Autodesk Fusion 360 part; units mm, degrees
(part 18 of 25)
  arc A5421 (73.9284, 22.9292) -> (73.8069, 23.2226) centre (73.8676, 23.0759) ccw
  line L1960 (79.2155, 20.3327) -> (79.2246, 20.3106)
  line L1961 (74.5699, 19.5453) -> (75.2188, 19.8141)
  arc A5422 (73.3311, 22.6949) -> (73.1066, 22.9194) centre (73.2189, 22.8072) ccw
  arc A5423 (73.8677, 23.2346) -> (73.8677, 22.9171) centre (73.8677, 23.0758) ccw
  arc A5424 (71.3073, 21.6383) -> (71.6007, 21.5168) centre (71.454, 21.5776) ccw
  arc A5425 (75.5687, 20.3714) -> (75.862, 20.2499) centre (75.7154, 20.3106) ccw
  line L1962 (71.628, 21.9976) -> (71.628, 24.4198)
  arc A5426 (81.0116, 19.692) -> (81.1331, 19.3986) centre (81.0724, 19.5453) ccw
  arc A5427 (72.6123, 21.6617) -> (72.2948, 21.6617) centre (72.4536, 21.6617) ccw
  arc A5428 (74.5699, 22.9171) -> (74.5699, 23.2346) centre (74.5699, 23.0758) ccw
  line L1963 (81.0723, 19.5453) -> (81.292, 19.6363)
  arc A5429 (73.1581, 18.4326) -> (73.2796, 18.1393) centre (73.2189, 18.2859) ccw
  arc A5430 (75.8712, 20.272) -> (75.5778, 20.3934) centre (75.7245, 20.3327) ccw
  arc A5431 (72.39, 25.2413) -> (72.39, 25.5588) centre (72.39, 25.4001) ccw
  arc A5432 (73.0125, 26.7442) -> (72.788, 26.5196) centre (72.9002, 26.6319) ccw
  arc A5433 (74.9617, 29.4567) -> (74.6442, 29.4567) centre (74.8029, 29.4567) ccw
  line L1964 (71.8797, 24.1681) -> (72.39, 24.1681)
  arc A5434 (71.7747, 21.9369) -> (71.4813, 22.0584) centre (71.628, 21.9977) ccw
  arc A5435 (72.2312, 24.1681) -> (72.5487, 24.1681) centre (72.3899, 24.1681) ccw
  arc A5436 (73.7806, 25.9103) -> (73.4631, 25.9103) centre (73.6218, 25.9103) ccw
  arc A5437 (73.9284, 18.408) -> (73.8069, 18.7014) centre (73.8676, 18.5547) ccw
  arc A5438 (79.2554, 18.0447) -> (79.4799, 17.8201) centre (79.3676, 17.9324) ccw
  arc A5439 (73.5177, 27.2925) -> (73.2002, 27.2925) centre (73.359, 27.2925) ccw
  arc A5440 (72.2312, 25.4) -> (72.5487, 25.4) centre (72.3899, 25.4) ccw
  arc A5441 (71.8797, 26.7906) -> (71.8797, 26.4731) centre (71.8797, 26.6319) ccw
  line L1965 (72.8653, 17.9324) -> (71.314, 17.9324)
  arc A5442 (74.6442, 28.9826) -> (74.9617, 28.9826) centre (74.8029, 28.9826) ccw
  arc A5443 (80.4308, 18.408) -> (80.3093, 18.7014) centre (80.3701, 18.5547) ccw
  arc A5444 (79.6605, 18.4326) -> (79.782, 18.1393) centre (79.7212, 18.2859) ccw
  line L1966 (72.39, 24.1681) -> (72.9003, 24.1681)
  arc A5445 (71.314, 18.0911) -> (71.314, 17.7736) centre (71.314, 17.9323) ccw
  arc A5446 (69.9162, 19.5548) -> (69.6917, 19.3303) centre (69.804, 19.4426) ccw
  line L1967 (74.803, 29.4567) -> (74.93, 29.5837)
  arc A5447 (72.5487, 26.6319) -> (72.2312, 26.6319) centre (72.3899, 26.6319) ccw
  arc A5448 (71.4692, 21.9976) -> (71.7867, 21.9976) centre (71.6279, 21.9976) ccw
  arc A5449 (75.0423, 29.4714) -> (74.8177, 29.6959) centre (74.93, 29.5837) ccw
  line L1968 (74.93, 29.5837) -> (75.2, 29.3137)
  arc A5450 (72.39, 24.3269) -> (72.39, 24.0094) centre (72.39, 24.1682) ccw
  arc A5451 (71.7867, 24.4198) -> (71.4692, 24.4198) centre (71.6279, 24.4198) ccw
  line L1969 (71.314, 17.9324) -> (69.8039, 19.4425)
  arc A5452 (74.5699, 18.3959) -> (74.5699, 18.7134) centre (74.5699, 18.5547) ccw
  arc A5453 (75.158, 18.1393) -> (75.2795, 18.4326) centre (75.2188, 18.2859) ccw
  arc A5454 (73.7342, 24.7775) -> (73.5096, 25.002) centre (73.6219, 24.8897) ccw
  arc A5455 (71.4692, 26.3802) -> (71.7867, 26.3802) centre (71.6279, 26.3802) ccw
  line L1970 (74.803, 28.9826) -> (74.803, 29.4567)
  line L1971 (71.628, 26.3802) -> (71.628, 26.797)
  line L1972 (71.454, 21.5775) -> (71.628, 21.9976)
  line L1973 (75.2188, 18.2859) -> (74.5699, 18.5547)
  line L1974 (72.9003, 26.6319) -> (72.39, 26.6319)
  arc A5456 (79.3677, 17.7736) -> (79.3677, 18.0911) centre (79.3677, 17.9323) ccw
  arc A5457 (72.9003, 24.0094) -> (72.9003, 24.3269) centre (72.9003, 24.1682) ccw
  arc A5458 (71.2018, 17.8201) -> (71.4263, 18.0447) centre (71.3141, 17.9324) ccw
  arc A5459 (69.6917, 19.5548) -> (69.9162, 19.3303) centre (69.804, 19.4426) ccw
  line L1975 (72.39, 24.1681) -> (72.39, 25.4)
  line L1976 (70.0659, 20.1895) -> (71.454, 21.5775)
  line L1977 (71.8797, 26.6319) -> (71.628, 26.3802)
  arc A5460 (74.9497, 28.9219) -> (74.6563, 29.0434) centre (74.803, 28.9827) ccw
  line L1978 (79.7212, 18.2859) -> (79.3677, 17.9324)
  line L1979 (72.39, 26.6319) -> (72.39, 25.4)
  arc A5461 (72.753, 18.0447) -> (72.9775, 17.8201) centre (72.8653, 17.9324) ccw
  arc A5462 (70.1781, 19.5923) -> (69.9536, 19.8168) centre (70.0658, 19.7046) ccw
  arc A5463 (69.9536, 20.3017) -> (70.1781, 20.0772) centre (70.0659, 20.1895) ccw
  arc A5464 (71.5662, 21.4653) -> (71.3417, 21.6898) centre (71.454, 21.5776) ccw
  arc A5465 (70.2246, 20.1895) -> (69.9071, 20.1895) centre (70.0658, 20.1895) ccw
  arc A5466 (72.2313, 25.4) -> (72.5488, 25.4) centre (72.3901, 25.4) ccw
  arc A5467 (79.8335, 18.1737) -> (79.609, 18.3982) centre (79.7212, 18.2859) ccw
  arc A5468 (74.4823, 28.6233) -> (74.7757, 28.5018) centre (74.629, 28.5626) ccw
  line L1980 (73.6219, 25.4) -> (72.39, 25.4)
  arc A5469 (72.9003, 26.4731) -> (72.9003, 26.7906) centre (72.9003, 26.6319) ccw
  arc A5470 (73.4712, 27.1803) -> (73.2467, 27.4048) centre (73.359, 27.2926) ccw
  arc A5471 (73.0982, 26.8243) -> (72.9767, 27.1177) centre (73.0375, 26.971) ccw
  arc A5472 (73.8677, 18.7134) -> (73.8677, 18.3959) centre (73.8677, 18.5547) ccw
  arc A5473 (75.4601, 17.8201) -> (75.6846, 18.0447) centre (75.5724, 17.9324) ccw
  arc A5474 (80.3701, 18.7134) -> (80.3701, 18.3959) centre (80.3701, 18.5547) ccw
  arc A5475 (75.5723, 18.0911) -> (75.5723, 17.7736) centre (75.5723, 17.9323) ccw
  line L1981 (72.39, 25.4) -> (73.6219, 25.4)
  line L1982 (75.5723, 17.9324) -> (75.2188, 18.2859)
  line L1983 (77.47, 29.5837) -> (77.74, 29.3137)
  line L1984 (77.74, 29.3137) -> (78.3889, 29.0449)
  line L1985 (80.2955, 29.6574) -> (80.4879, 29.5176)
  arc A5476 (80.1832, 29.5452) -> (80.4077, 29.7697) centre (80.2955, 29.6575) ccw
  arc A5477 (78.3281, 28.8982) -> (78.4496, 29.1916) centre (78.3889, 29.0449) ccw
  line L1986 (81.28, 29.2989) -> (81.28, 31.75)
  arc A5478 (72.39, 26.4731) -> (72.39, 26.7906) centre (72.39, 26.6319) ccw
  arc A5479 (73.4631, 24.8897) -> (73.7806, 24.8897) centre (73.6218, 24.8897) ccw
  line L1987 (75.8489, 29.0449) -> (76.5511, 29.0449)
  arc A5480 (72.39, 25.5588) -> (72.39, 25.2413) centre (72.39, 25.4001) ccw
  arc A5481 (73.4631, 25.4) -> (73.7806, 25.4) centre (73.6218, 25.4) ccw
  arc A5482 (72.39, 26.7906) -> (72.39, 26.4731) centre (72.39, 26.6319) ccw
  arc A5483 (73.6219, 25.2413) -> (73.6219, 25.5588) centre (73.6219, 25.4001) ccw
  arc A5484 (77.6278, 29.2014) -> (77.8523, 29.4259) centre (77.74, 29.3136) ccw
  arc A5485 (71.628, 26.9558) -> (71.628, 26.6382) centre (71.628, 26.797) ccw
  line L1988 (74.629, 28.5625) -> (74.803, 28.9826)
  line L1989 (76.5511, 29.0449) -> (77.2, 29.3137)
  arc A5486 (77.8008, 29.4603) -> (77.6793, 29.167) centre (77.74, 29.3137) ccw
  arc A5487 (79.0304, 29.1916) -> (79.1519, 28.8982) centre (79.0911, 29.0449) ccw
  arc A5488 (73.6219, 25.2412) -> (73.6219, 25.5587) centre (73.6219, 25.4) ccw
  arc A5489 (81.28, 31.9087) -> (81.28, 31.5912) centre (81.28, 31.75) ccw
  arc A5490 (81.1362, 29.1421) -> (81.1859, 29.4557) centre (81.1611, 29.2989) ccw
  arc A5491 (72.788, 24.2804) -> (73.0125, 24.0558) centre (72.9003, 24.1681) ccw
  arc A5492 (72.39, 25.5587) -> (72.39, 25.2412) centre (72.39, 25.4) ccw
  arc A5493 (72.39, 25.5588) -> (72.39, 25.2413) centre (72.39, 25.4001) ccw
  arc A5494 (71.7867, 26.797) -> (71.4692, 26.797) centre (71.6279, 26.797) ccw
  arc A5495 (73.2002, 27.2925) -> (73.5177, 27.2925) centre (73.359, 27.2925) ccw
  line L1990 (79.0911, 29.0449) -> (79.74, 29.3137)
  arc A5496 (78.3889, 29.2037) -> (78.3889, 28.8862) centre (78.3889, 29.045) ccw
  arc A5497 (81.1212, 29.2989) -> (81.4387, 29.2989) centre (81.2799, 29.2989) ccw
  arc A5498 (75.0423, 29.6959) -> (74.8177, 29.4714) centre (74.93, 29.5836) ccw
  line L1991 (81.28, 31.75) -> (81.28, 29.2989)
  arc A5499 (81.4388, 31.75) -> (81.1213, 31.75) centre (81.2801, 31.75) ccw
  arc A5500 (75.7881, 28.8982) -> (75.9096, 29.1916) centre (75.8488, 29.0449) ccw
  arc A5501 (74.7412, 28.4503) -> (74.5167, 28.6748) centre (74.629, 28.5626) ccw
  arc A5502 (74.6907, 29.5689) -> (74.9153, 29.3444) centre (74.803, 29.4566) ccw
  line L1992 (72.39, 25.4) -> (72.39, 26.6319)
  arc A5503 (81.1611, 29.4577) -> (81.1611, 29.1401) centre (81.1611, 29.2989) ccw
  arc A5504 (71.992, 26.5196) -> (71.7675, 26.7441) centre (71.8798, 26.6319) ccw
  arc A5505 (71.5157, 26.4924) -> (71.7403, 26.2679) centre (71.628, 26.3802) ccw
  arc A5506 (73.5096, 25.798) -> (73.7342, 26.0225) centre (73.6219, 25.9103) ccw
  line L1993 (72.9003, 24.1681) -> (73.6219, 24.8897)
  arc A5507 (72.5488, 26.6319) -> (72.2313, 26.6319) centre (72.3901, 26.6319) ccw
  arc A5508 (81.28, 31.5912) -> (81.28, 31.9087) centre (81.28, 31.75) ccw
  arc A5509 (73.2467, 27.4048) -> (73.4712, 27.1803) centre (73.359, 27.2926) ccw
  line L1994 (73.359, 27.2925) -> (74.629, 28.5625)
  arc A5510 (72.6174, 26.6382) -> (72.6174, 26.9558) centre (72.6174, 26.797) ccw
  line L1995 (73.6219, 25.4) -> (73.6219, 25.9103)
  arc A5511 (72.5566, 26.9437) -> (72.6781, 26.6503) centre (72.6174, 26.797) ccw
  arc A5512 (72.9252, 27.0833) -> (73.1497, 26.8588) centre (73.0375, 26.9711) ccw
  line L1996 (80.9261, 29.3361) -> (81.1611, 29.2989)
  line L1997 (73.0375, 26.971) -> (73.359, 27.2925)
  line L1998 (71.628, 26.797) -> (72.6174, 26.797)
  arc A5513 (73.7806, 25.4) -> (73.4631, 25.4) centre (73.6218, 25.4) ccw
  line L1999 (73.6219, 24.8897) -> (73.6219, 25.4)
  arc A5514 (72.5488, 25.4) -> (72.2313, 25.4) centre (72.3901, 25.4) ccw
  arc A5515 (72.2313, 25.4) -> (72.5488, 25.4) centre (72.3901, 25.4) ccw
  arc A5516 (80.3019, 29.8755) -> (80.0773, 29.651) centre (80.1896, 29.7633) ccw
  line L2000 (80.1896, 29.7633) -> (80.2955, 29.6574)
  arc A5517 (80.3888, 29.7859) -> (80.2021, 29.529) centre (80.2954, 29.6575) ccw
  line L2001 (73.6219, 25.9103) -> (72.9003, 26.6319)
  line L2002 (72.6174, 26.797) -> (73.0375, 26.971)
  line L2003 (72.39, 26.6319) -> (71.8797, 26.6319)
  arc A5518 (77.5823, 29.6959) -> (77.3577, 29.4714) centre (77.47, 29.5837) ccw
  arc A5519 (82.9051, 30.4072) -> (82.6031, 30.5054) centre (82.7541, 30.4563) ccw
  line L2004 (81.28, 29.2989) -> (81.3989, 29.2989)
  arc A5520 (81.1213, 29.2989) -> (81.4388, 29.2989) centre (81.2801, 29.2989) ccw
  arc A5521 (81.9092, 29.2586) -> (81.8111, 29.5606) centre (81.8602, 29.4096) ccw
  line L2005 (81.3989, 29.2989) -> (81.6339, 29.3361)
  arc A5522 (81.3989, 29.1401) -> (81.3989, 29.4577) centre (81.3989, 29.2989) ccw
  arc A5523 (79.6277, 29.4259) -> (79.8522, 29.2014) centre (79.74, 29.3137) ccw
  line L2006 (81.1611, 29.2989) -> (81.28, 29.2989)
  arc A5524 (80.6278, 29.2682) -> (80.7719, 29.5511) centre (80.6998, 29.4097) ccw
  arc A5525 (75.2608, 29.4603) -> (75.1393, 29.167) centre (75.2001, 29.3137) ccw
  arc A5526 (81.4388, 31.75) -> (81.1213, 31.75) centre (81.2801, 31.75) ccw
  arc A5527 (82.4441, 33.3886) -> (82.701, 33.5752) centre (82.5726, 33.4819) ccw
  arc A5528 (81.6091, 34.0071) -> (81.6587, 34.3207) centre (81.6339, 34.1639) ccw
  line L2007 (82.7541, 33.0437) -> (82.6806, 33.2699)
  arc A5529 (80.877, 29.1851) -> (80.9752, 29.4871) centre (80.9261, 29.3361) ccw
  arc A5530 (77.2607, 29.167) -> (77.1392, 29.4603) centre (77.2, 29.3137) ccw
  arc A5531 (81.4387, 31.75) -> (81.1212, 31.75) centre (81.2799, 31.75) ccw
  arc A5532 (81.28, 34.3598) -> (81.28, 34.0423) centre (81.28, 34.2011) ccw
  arc A5533 (82.95, 32.8087) -> (82.6325, 32.8087) centre (82.7913, 32.8087) ccw
  arc A5534 (81.7881, 29.5511) -> (81.9322, 29.2682) centre (81.8602, 29.4096) ccw
  arc A5535 (82.4311, 30.0902) -> (82.714, 29.946) centre (82.5725, 30.0181) ccw
  arc A5536 (80.3019, 29.651) -> (80.0773, 29.8755) centre (80.1896, 29.7633) ccw
  arc A5537 (82.545, 29.7134) -> (82.3205, 29.9379) centre (82.4327, 29.8257) ccw
  line L2008 (81.6339, 34.1639) -> (81.3989, 34.2011)
  arc A5538 (79.8007, 29.167) -> (79.6792, 29.4603) centre (79.74, 29.3137) ccw
  arc A5539 (76.5511, 28.8862) -> (76.5511, 29.2037) centre (76.5511, 29.045) ccw
  arc A5540 (81.3741, 29.4557) -> (81.4238, 29.1421) centre (81.399, 29.2989) ccw
  arc A5541 (80.56, 29.6591) -> (80.4158, 29.3762) centre (80.4879, 29.5177) ccw
  line L2009 (82.4328, 33.6743) -> (82.2645, 33.8426)
  line L2010 (82.7913, 31.75) -> (81.28, 31.75)
  line L2011 (82.7913, 32.8087) -> (82.7541, 33.0437)
  arc A5542 (81.28, 31.9088) -> (81.28, 31.5913) centre (81.28, 31.7501) ccw
  line L2012 (82.6806, 33.2699) -> (82.5726, 33.4819)
  arc A5543 (77.0877, 29.4259) -> (77.3122, 29.2014) centre (77.2, 29.3136) ccw
  line L2013 (79.74, 29.3137) -> (80.1896, 29.7633)
  arc A5544 (81.28, 29.1401) -> (81.28, 29.4577) centre (81.28, 29.2989) ccw
  arc A5545 (80.7489, 29.5606) -> (80.6508, 29.2586) centre (80.6999, 29.4096) ccw
  line L2014 (75.2, 29.3137) -> (75.8489, 29.0449)
  arc A5546 (75.8489, 29.2037) -> (75.8489, 28.8862) centre (75.8489, 29.045) ccw
  arc A5547 (81.4238, 34.3579) -> (81.3741, 34.0443) centre (81.399, 34.2011) ccw
  line L2015 (80.4879, 29.5176) -> (80.6999, 29.4096)
  arc A5548 (76.4904, 29.1916) -> (76.6119, 28.8982) centre (76.5512, 29.0449) ccw
  line L2016 (82.2645, 29.6574) -> (82.4328, 29.8257)
  line L2017 (81.3989, 34.2011) -> (81.28, 34.2011)
  arc A5549 (82.5612, 33.7677) -> (82.3043, 33.581) centre (82.4327, 33.6744) ccw
  arc A5550 (82.714, 33.554) -> (82.4311, 33.4098) centre (82.5726, 33.4819) ccw
  line L2018 (80.6999, 29.4096) -> (80.9261, 29.3361)
  arc A5551 (80.9509, 29.4929) -> (80.9013, 29.1793) centre (80.9261, 29.3361) ccw
  line L2019 (82.0721, 33.9824) -> (81.8601, 34.0904)
  arc A5552 (79.0911, 28.8862) -> (79.0911, 29.2037) centre (79.0911, 29.045) ccw
  line L2020 (81.8601, 29.4096) -> (82.0721, 29.5176)
  arc A5553 (77.5823, 29.4714) -> (77.3577, 29.6959) centre (77.47, 29.5837) ccw
  arc A5554 (81.28, 29.4577) -> (81.28, 29.1401) centre (81.28, 29.2989) ccw
  arc A5555 (81.6587, 29.1793) -> (81.6091, 29.4929) centre (81.6339, 29.3361) ccw
  arc A5556 (82.8316, 33.319) -> (82.5296, 33.2209) centre (82.6806, 33.27) ccw
  arc A5557 (82.6325, 30.6913) -> (82.95, 30.6913) centre (82.7913, 30.6913) ccw
  arc A5558 (82.5391, 33.1979) -> (82.822, 33.342) centre (82.6806, 33.27) ccw
  arc A5559 (82.3043, 29.919) -> (82.5612, 29.7323) centre (82.4327, 29.8256) ccw
  arc A5560 (80.3946, 29.3892) -> (80.5812, 29.646) centre (80.4879, 29.5176) ccw
  line L2021 (81.6339, 29.3361) -> (81.8601, 29.4096)
  line L2022 (77.2, 29.3137) -> (77.47, 29.5837)
  arc A5561 (75.0878, 29.2014) -> (75.3123, 29.4259) centre (75.2001, 29.3137) ccw
  line L2023 (78.3889, 29.0449) -> (79.0911, 29.0449)
  arc A5562 (81.5848, 29.4871) -> (81.683, 29.1851) centre (81.6339, 29.3361) ccw
  arc A5563 (81.28, 31.9087) -> (81.28, 31.5912) centre (81.28, 31.75) ccw
  line L2024 (82.6806, 30.2301) -> (82.7541, 30.4563)
  arc A5564 (79.7786, 34.3422) -> (79.6572, 34.0488) centre (79.7179, 34.1955) ccw
  arc A5565 (82.3768, 33.9548) -> (82.1523, 33.7303) centre (82.2646, 33.8425) ccw
  line L2025 (80.6999, 34.0904) -> (80.4879, 33.9824)
  arc A5566 (81.4387, 44.45) -> (81.1212, 44.45) centre (81.2799, 44.45) ccw
  line L2026 (80.4879, 33.9824) -> (80.2955, 33.8426)
  arc A5567 (82, 33.8409) -> (82.1442, 34.1238) centre (82.0721, 33.9824) ccw
  arc A5568 (81.4388, 34.2011) -> (81.1213, 34.2011) centre (81.2801, 34.2011) ccw
  arc A5569 (80.3888, 42.4859) -> (80.2021, 42.229) centre (80.2954, 42.3575) ccw
  arc A5570 (81.1213, 31.75) -> (81.4388, 31.75) centre (81.2801, 31.75) ccw
  arc A5571 (80.0773, 33.6244) -> (80.3019, 33.849) centre (80.1896, 33.7367) ccw
  line L2027 (82.2645, 33.8426) -> (82.0721, 33.9824)
  line L2028 (82.5726, 30.0181) -> (82.6806, 30.2301)
  arc A5572 (82.701, 29.9248) -> (82.4441, 30.1114) centre (82.5726, 30.0181) ccw
  line L2029 (82.5726, 33.4819) -> (82.4328, 33.6743)
  arc A5573 (81.1611, 42.1576) -> (81.1611, 41.8402) centre (81.1611, 41.9989) ccw
  arc A5574 (82.5296, 30.2791) -> (82.8316, 30.181) centre (82.6806, 30.23) ccw
  line L2030 (82.7541, 30.4563) -> (82.7913, 30.6913)
  line L2031 (82.7913, 30.6913) -> (82.7913, 31.75)
  arc A5575 (82.3205, 33.5621) -> (82.545, 33.7866) centre (82.4327, 33.6743) ccw
  arc A5576 (81.9322, 34.2318) -> (81.7881, 33.9489) centre (81.8602, 34.0903) ccw
  arc A5577 (81.9788, 29.646) -> (82.1654, 29.3892) centre (82.0721, 29.5176) ccw
  arc A5578 (82.95, 31.75) -> (82.6325, 31.75) centre (82.7913, 31.75) ccw
  line L2032 (81.28, 31.75) -> (82.7913, 31.75)
  arc A5579 (82.1442, 29.3762) -> (82, 29.6591) centre (82.0721, 29.5176) ccw
  arc A5580 (82.5973, 30.4811) -> (82.9109, 30.4315) centre (82.7541, 30.4563) ccw
  arc A5581 (82.9481, 30.6664) -> (82.6345, 30.7161) centre (82.7913, 30.6913) ccw
  arc A5582 (82.7913, 31.5913) -> (82.7913, 31.9088) centre (82.7913, 31.7501) ccw
  line L2033 (82.4328, 29.8257) -> (82.5726, 30.0181)
  arc A5583 (82.7913, 31.5912) -> (82.7913, 31.9087) centre (82.7913, 31.75) ccw
  line L2034 (81.8601, 34.0904) -> (81.6339, 34.1639)
  line L2035 (82.7913, 31.75) -> (82.7913, 32.8087)
  arc A5584 (82.822, 30.158) -> (82.5391, 30.3021) centre (82.6806, 30.2301) ccw
  arc A5585 (82.6031, 32.9946) -> (82.9051, 33.0928) centre (82.7541, 33.0437) ccw
  arc A5586 (81.683, 34.3149) -> (81.5848, 34.0129) centre (81.6339, 34.1639) ccw
  arc A5587 (82.1712, 33.7141) -> (82.3579, 33.971) centre (82.2646, 33.8426) ccw
  arc A5588 (81.1213, 31.75) -> (81.4388, 31.75) centre (81.2801, 31.75) ccw
  arc A5589 (79.6277, 42.1259) -> (79.8522, 41.9014) centre (79.74, 42.0137) ccw
  arc A5590 (81.1212, 41.9989) -> (81.4387, 41.9989) centre (81.2799, 41.9989) ccw
  arc A5591 (81.28, 44.2912) -> (81.28, 44.6087) centre (81.28, 44.4499) ccw
  line L2036 (80.1896, 42.4633) -> (80.2955, 42.3574)
  arc A5592 (82.6325, 31.75) -> (82.95, 31.75) centre (82.7913, 31.75) ccw
  line L2037 (81.28, 34.2011) -> (81.1611, 34.2011)
  line L2038 (80.2955, 33.8426) -> (80.1896, 33.7367)
  arc A5593 (82.1654, 34.1108) -> (81.9788, 33.8539) centre (82.0721, 33.9824) ccw
  arc A5594 (82.3579, 29.529) -> (82.1712, 29.7859) centre (82.2646, 29.6575) ccw
  line L2039 (80.1896, 33.7367) -> (79.74, 34.1863)
  arc A5595 (81.1212, 31.75) -> (81.4387, 31.75) centre (81.2799, 31.75) ccw
  arc A5596 (80.6508, 34.2414) -> (80.7489, 33.9394) centre (80.6999, 34.0904) ccw
  arc A5597 (80.9752, 34.0129) -> (80.877, 34.3149) centre (80.9261, 34.1639) ccw
  arc A5598 (82.6345, 32.7839) -> (82.9481, 32.8336) centre (82.7913, 32.8088) ccw
  arc A5599 (81.8111, 33.9394) -> (81.9092, 34.2414) centre (81.8602, 34.0904) ccw
  arc A5600 (80.5812, 33.8539) -> (80.3946, 34.1108) centre (80.4879, 33.9824) ccw
  arc A5601 (79.5591, 34.1955) -> (79.8766, 34.1955) centre (79.7178, 34.1955) ccw
  line L2040 (79.7179, 42.0045) -> (79.74, 42.0137)
  line L2041 (82.0721, 29.5176) -> (82.2645, 29.6574)
  arc A5602 (82.9109, 33.0685) -> (82.5973, 33.0189) centre (82.7541, 33.0437) ccw
  arc A5603 (80.3019, 42.351) -> (80.0773, 42.5755) centre (80.1896, 42.4633) ccw
  line L2042 (80.4879, 42.2176) -> (80.6999, 42.1096)
  arc A5604 (82.1523, 29.7697) -> (82.3768, 29.5452) centre (82.2646, 29.6575) ccw
  line L2043 (81.28, 34.2011) -> (81.28, 31.75)
  arc A5605 (81.1859, 34.0443) -> (81.1362, 34.3579) centre (81.1611, 34.2011) ccw
  arc A5606 (80.3946, 42.0892) -> (80.5812, 42.346) centre (80.4879, 42.2176) ccw
  arc A5607 (80.877, 41.8851) -> (80.9752, 42.1871) centre (80.9261, 42.0361) ccw
  arc A5608 (81.1362, 41.8421) -> (81.1859, 42.1557) centre (81.1611, 41.9989) ccw
  line L2044 (82.7541, 43.1563) -> (82.7913, 43.3913)
  line L2045 (81.28, 41.9989) -> (81.28, 44.45)
  line L2046 (81.28, 41.9989) -> (81.3989, 41.9989)
  line L2047 (79.74, 34.1863) -> (79.7179, 34.1955)
  arc A5609 (79.6792, 34.0397) -> (79.8007, 34.333) centre (79.74, 34.1864) ccw
  arc A5610 (80.56, 42.3591) -> (80.4158, 42.0762) centre (80.4879, 42.2177) ccw
  arc A5611 (81.28, 41.8402) -> (81.28, 42.1576) centre (81.28, 41.9989) ccw
  line L2048 (80.2955, 42.3574) -> (80.4879, 42.2176)
  line L2049 (80.9261, 34.1639) -> (80.6999, 34.0904)
  line L2050 (82.7913, 45.5087) -> (82.7541, 45.7437)
  arc A5612 (80.7719, 33.9489) -> (80.6278, 34.2318) centre (80.6998, 34.0904) ccw
  arc A5613 (80.4077, 33.7303) -> (80.1832, 33.9548) centre (80.2955, 33.8425) ccw
  arc A5614 (79.6572, 42.1512) -> (79.7786, 41.8578) centre (79.7179, 42.0045) ccw
  arc A5615 (79.8766, 42.0045) -> (79.5591, 42.0045) centre (79.7178, 42.0045) ccw
  arc A5616 (81.28, 31.9088) -> (81.28, 31.5913) centre (81.28, 31.7501) ccw
  arc A5617 (80.0773, 33.849) -> (80.3019, 33.6244) centre (80.1896, 33.7367) ccw
  arc A5618 (79.8522, 34.2986) -> (79.6277, 34.0741) centre (79.74, 34.1864) ccw
  arc A5619 (80.2021, 33.971) -> (80.3888, 33.7141) centre (80.2954, 33.8426) ccw
  arc A5620 (80.1832, 42.2452) -> (80.4077, 42.4697) centre (80.2955, 42.3575) ccw
  arc A5621 (80.4158, 34.1238) -> (80.56, 33.8409) centre (80.4879, 33.9824) ccw
  line L2051 (81.28, 44.45) -> (81.28, 41.9989)
  arc A5622 (81.28, 31.5913) -> (81.28, 31.9088) centre (81.28, 31.7501) ccw
  arc A5623 (81.1611, 34.3598) -> (81.1611, 34.0423) centre (81.1611, 34.2011) ccw
  arc A5624 (82.5612, 46.4677) -> (82.3043, 46.281) centre (82.4327, 46.3743) ccw
  arc A5625 (80.3019, 42.5755) -> (80.0773, 42.351) centre (80.1896, 42.4633) ccw
  arc A5626 (79.8007, 41.867) -> (79.6792, 42.1603) centre (79.7399, 42.0136) ccw
  line L2052 (82.4328, 46.3743) -> (82.2645, 46.5426)
  arc A5627 (82.6031, 45.6946) -> (82.9051, 45.7928) centre (82.7541, 45.7437) ccw
  arc A5628 (82.5973, 43.1811) -> (82.9109, 43.1315) centre (82.7541, 43.1563) ccw
  line L2053 (82.5726, 46.1819) -> (82.4328, 46.3743)
  line L2054 (79.7179, 34.1955) -> (79.7179, 42.0045)
  arc A5629 (80.6278, 41.9682) -> (80.7719, 42.2511) centre (80.6998, 42.1097) ccw
  arc A5630 (80.9013, 34.3207) -> (80.9509, 34.0071) centre (80.9261, 34.1639) ccw
  line L2055 (80.9261, 42.0361) -> (81.1611, 41.9989)
  arc A5631 (82.95, 44.45) -> (82.6325, 44.45) centre (82.7913, 44.45) ccw
  arc A5632 (81.4387, 34.2011) -> (81.1212, 34.2011) centre (81.2799, 34.2011) ccw
  arc A5633 (82.3205, 46.2621) -> (82.545, 46.4866) centre (82.4327, 46.3743) ccw
  arc A5634 (80.9509, 42.1929) -> (80.9013, 41.8793) centre (80.9261, 42.0361) ccw
  line L2056 (82.2645, 46.5426) -> (82.0721, 46.6824)
  line L2057 (79.74, 42.0137) -> (80.1896, 42.4633)
  line L2058 (81.1611, 34.2011) -> (80.9261, 34.1639)
  arc A5635 (82.8316, 46.019) -> (82.5296, 45.9209) centre (82.6806, 45.9699) ccw
  arc A5636 (82.1442, 42.0762) -> (82, 42.3591) centre (82.0721, 42.2177) ccw
  line L2059 (82.5726, 42.7181) -> (82.6806, 42.9301)
  line L2060 (81.28, 44.45) -> (82.7913, 44.45)
  line L2061 (81.6339, 42.0361) -> (81.8601, 42.1096)
  arc A5637 (81.5848, 42.1871) -> (81.683, 41.8851) centre (81.6339, 42.0361) ccw
  arc A5638 (80.7489, 42.2606) -> (80.6508, 41.9586) centre (80.6999, 42.1096) ccw
  line L2062 (82.6806, 45.9699) -> (82.5726, 46.1819)
  arc A5639 (82.4441, 46.0886) -> (82.701, 46.2752) centre (82.5726, 46.1819) ccw
  arc A5640 (81.28, 34.0423) -> (81.28, 34.3598) centre (81.28, 34.2011) ccw
  line L2063 (81.1611, 41.9989) -> (81.28, 41.9989)
  arc A5641 (82.3768, 46.6548) -> (82.1523, 46.4303) centre (82.2646, 46.5425) ccw
  arc A5642 (82.7913, 44.2913) -> (82.7913, 44.6088) centre (82.7913, 44.4501) ccw
  line L2064 (80.6999, 42.1096) -> (80.9261, 42.0361)
  arc A5643 (81.3989, 34.0423) -> (81.3989, 34.3598) centre (81.3989, 34.2011) ccw
  arc A5644 (81.6587, 41.8793) -> (81.6091, 42.1929) centre (81.6339, 42.0361) ccw
  arc A5645 (82.6325, 44.45) -> (82.95, 44.45) centre (82.7913, 44.45) ccw
  arc A5646 (82.545, 42.4134) -> (82.3205, 42.6379) centre (82.4327, 42.5257) ccw
  arc A5647 (81.1213, 44.45) -> (81.4388, 44.45) centre (81.2801, 44.45) ccw
  line L2065 (81.28, 31.75) -> (81.28, 34.2011)
  arc A5648 (82.95, 45.5087) -> (82.6325, 45.5087) centre (82.7913, 45.5087) ccw
  line L2066 (81.28, 46.9011) -> (81.28, 44.45)
  arc A5649 (81.1213, 41.9989) -> (81.4388, 41.9989) centre (81.2801, 41.9989) ccw
  arc A5650 (82.1523, 42.4697) -> (82.3768, 42.2452) centre (82.2646, 42.3575) ccw
  arc A5651 (82.3579, 42.229) -> (82.1712, 42.4859) centre (82.2646, 42.3575) ccw
  arc A5652 (81.4388, 44.45) -> (81.1213, 44.45) centre (81.2801, 44.45) ccw
  line L2067 (82.7541, 45.7437) -> (82.6806, 45.9699)
  arc A5653 (81.28, 42.1576) -> (81.28, 41.8402) centre (81.28, 41.9989) ccw
  arc A5654 (81.3989, 41.8402) -> (81.3989, 42.1576) centre (81.3989, 41.9989) ccw
  arc A5655 (82.7913, 44.2912) -> (82.7913, 44.6087) centre (82.7913, 44.4499) ccw
  line L2068 (82.0721, 42.2176) -> (82.2645, 42.3574)
  arc A5656 (82.6325, 43.3913) -> (82.95, 43.3913) centre (82.7913, 43.3913) ccw
  arc A5657 (82.9481, 43.3664) -> (82.6345, 43.4161) centre (82.7913, 43.3912) ccw
  arc A5658 (82.9051, 43.1072) -> (82.6031, 43.2054) centre (82.7541, 43.1563) ccw
  arc A5659 (82.714, 46.254) -> (82.4311, 46.1098) centre (82.5725, 46.1819) ccw
  arc A5660 (82.4311, 42.7902) -> (82.714, 42.646) centre (82.5725, 42.7181) ccw
  line L2069 (82.4328, 42.5257) -> (82.5726, 42.7181)
  line L2070 (82.2645, 42.3574) -> (82.4328, 42.5257)
  arc A5661 (81.9092, 41.9586) -> (81.8111, 42.2606) centre (81.8602, 42.1096) ccw
  arc A5662 (80.6508, 46.9414) -> (80.7489, 46.6394) centre (80.6999, 46.7904) ccw
  arc A5663 (77.3122, 46.9986) -> (77.0877, 46.7741) centre (77.2, 46.8863) ccw
  arc A5664 (77.1392, 46.7397) -> (77.2607, 47.033) centre (77.2, 46.8863) ccw
  arc A5665 (82.5296, 42.9791) -> (82.8316, 42.881) centre (82.6806, 42.9301) ccw
  arc A5666 (82.3043, 42.619) -> (82.5612, 42.4323) centre (82.4327, 42.5256) ccw
  arc A5667 (81.4388, 44.45) -> (81.1213, 44.45) centre (81.2801, 44.45) ccw
  arc A5668 (82.701, 42.6248) -> (82.4441, 42.8114) centre (82.5726, 42.7181) ccw
  line L2071 (82.7913, 44.45) -> (82.7913, 45.5087)
  arc A5669 (77.8523, 46.7741) -> (77.6278, 46.9986) centre (77.74, 46.8863) ccw
  line L2072 (77.2, 46.8863) -> (76.5511, 47.1551)
  arc A5670 (75.8489, 47.3138) -> (75.8489, 46.9963) centre (75.8489, 47.1551) ccw
  arc A5671 (76.5511, 46.9963) -> (76.5511, 47.3138) centre (76.5511, 47.1551) ccw
  arc A5672 (81.6091, 46.7071) -> (81.6587, 47.0207) centre (81.6339, 46.8639) ccw
  arc A5673 (82.1712, 46.4141) -> (82.3579, 46.671) centre (82.2646, 46.5425) ccw
  line L2073 (80.9261, 46.8639) -> (80.6999, 46.7904)
  arc A5674 (77.6793, 47.033) -> (77.8008, 46.7397) centre (77.74, 46.8863) ccw
  line L2074 (82.6806, 42.9301) -> (82.7541, 43.1563)
  arc A5675 (80.7719, 46.6489) -> (80.6278, 46.9318) centre (80.6998, 46.7904) ccw
  line L2075 (81.1611, 46.9011) -> (80.9261, 46.8639)
  line L2076 (81.8601, 42.1096) -> (82.0721, 42.2176)
  arc A5676 (82.9109, 45.7685) -> (82.5973, 45.7189) centre (82.7541, 45.7437) ccw
  arc A5677 (80.4077, 46.4303) -> (80.1832, 46.6548) centre (80.2955, 46.5426) ccw
  arc A5678 (81.28, 44.6088) -> (81.28, 44.2913) centre (81.28, 44.4501) ccw
  arc A5679 (81.4387, 46.9011) -> (81.1212, 46.9011) centre (81.2799, 46.9011) ccw
  arc A5680 (81.4238, 47.0579) -> (81.3741, 46.7443) centre (81.399, 46.9011) ccw
  arc A5681 (79.6792, 46.7397) -> (79.8007, 47.033) centre (79.7399, 46.8864) ccw
  arc A5682 (81.28, 44.6087) -> (81.28, 44.2912) centre (81.28, 44.4499) ccw
  arc A5683 (81.1611, 47.0598) -> (81.1611, 46.7423) centre (81.1611, 46.901) ccw
  line L2077 (82.0721, 46.6824) -> (81.8601, 46.7904)
  line L2078 (80.2955, 46.5426) -> (80.1896, 46.4367)
  line L2079 (79.0911, 47.1551) -> (78.3889, 47.1551)
  arc A5684 (81.8111, 46.6394) -> (81.9092, 46.9414) centre (81.8602, 46.7904) ccw
  arc A5685 (81.28, 47.0598) -> (81.28, 46.7423) centre (81.28, 46.901) ccw
  arc A5686 (79.0911, 46.9963) -> (79.0911, 47.3138) centre (79.0911, 47.1551) ccw
  arc A5687 (82.5391, 45.8979) -> (82.822, 46.042) centre (82.6806, 45.97) ccw
  arc A5688 (81.28, 44.6087) -> (81.28, 44.2912) centre (81.28, 44.4499) ccw
  arc A5689 (81.3741, 42.1557) -> (81.4238, 41.8421) centre (81.399, 41.9989) ccw
  arc A5690 (82.822, 42.858) -> (82.5391, 43.0021) centre (82.6806, 42.9301) ccw
  line L2080 (82.7913, 43.3913) -> (82.7913, 44.45)
  arc A5691 (82.1654, 46.8108) -> (81.9788, 46.5539) centre (82.0721, 46.6823) ccw
  arc A5692 (82.6345, 45.4839) -> (82.9481, 45.5336) centre (82.7913, 45.5088) ccw
  arc A5693 (81.7881, 42.2511) -> (81.9322, 41.9682) centre (81.8602, 42.1097) ccw
  arc A5694 (81.9788, 42.346) -> (82.1654, 42.0892) centre (82.0721, 42.2176) ccw
  line L2081 (81.3989, 41.9989) -> (81.6339, 42.0361)
  line L2082 (82.7913, 44.45) -> (81.28, 44.45)
  arc A5695 (79.8522, 46.9986) -> (79.6277, 46.7741) centre (79.74, 46.8864) ccw
  line L2083 (78.3889, 47.1551) -> (77.74, 46.8863)
  arc A5696 (74.93, 49.6887) -> (74.93, 49.3712) centre (74.93, 49.53) ccw
  line L2084 (80.1896, 46.4367) -> (79.74, 46.8863)
  arc A5697 (80.0773, 46.3244) -> (80.3019, 46.549) centre (80.1896, 46.4367) ccw
  arc A5698 (81.9322, 46.9318) -> (81.7881, 46.6489) centre (81.8602, 46.7903) ccw
  line L2085 (81.3989, 46.9011) -> (81.28, 46.9011)
  line L2086 (77.74, 46.8863) -> (77.47, 46.6163)
  arc A5699 (81.1212, 44.45) -> (81.4387, 44.45) centre (81.2799, 44.45) ccw
  arc A5700 (79.1519, 47.3018) -> (79.0304, 47.0084) centre (79.0911, 47.1551) ccw
  arc A5701 (78.4496, 47.0084) -> (78.3281, 47.3018) centre (78.3889, 47.1551) ccw
  line L2087 (74.93, 49.53) -> (76.3016, 49.53)
  arc A5702 (74.93, 51.0603) -> (74.93, 50.7428) centre (74.93, 50.9016) ccw
  arc A5703 (81.3989, 46.7423) -> (81.3989, 47.0598) centre (81.3989, 46.901) ccw
  arc A5704 (75.4981, 50.7428) -> (75.4981, 51.0603) centre (75.4981, 50.9016) ccw
  arc A5705 (74.93, 48.3171) -> (74.93, 47.9997) centre (74.93, 48.1584) ccw
  arc A5706 (76.1428, 48.9619) -> (76.4603, 48.9619) centre (76.3016, 48.9619) ccw
  arc A5707 (73.8413, 47.3138) -> (73.8413, 46.9963) centre (73.8413, 47.1551) ccw
  line L2088 (81.6339, 46.8639) -> (81.3989, 46.9011)
  arc A5708 (73.4207, 48.4863) -> (73.6453, 48.2618) centre (73.533, 48.3741) ccw
  line L2089 (74.0111, 47.1551) -> (73.8413, 47.1551)
  line L2090 (75.4981, 48.1584) -> (76.3016, 48.9619)
  arc A5709 (75.1393, 47.033) -> (75.2608, 46.7397) centre (75.2001, 46.8864) ccw
  line L2091 (73.533, 47.4634) -> (73.533, 48.3741)
  arc A5710 (74.93, 49.6888) -> (74.93, 49.3713) centre (74.93, 49.5301) ccw
  arc A5711 (80.5812, 46.5539) -> (80.3946, 46.8108) centre (80.4879, 46.6823) ccw
  arc A5712 (76.4603, 50.0981) -> (76.1428, 50.0981) centre (76.3016, 50.0981) ccw
  arc A5713 (75.0888, 49.53) -> (74.7713, 49.53) centre (74.93, 49.53) ccw
  line L2092 (80.4879, 46.6824) -> (80.2955, 46.5426)
  arc A5714 (76.4603, 49.53) -> (76.1428, 49.53) centre (76.3016, 49.53) ccw
  line L2093 (74.66, 46.8863) -> (74.0111, 47.1551)
  arc A5715 (75.6104, 51.0139) -> (75.3859, 50.7893) centre (75.4982, 50.9016) ccw
  line L2094 (77.47, 46.6163) -> (77.2, 46.8863)
  line L2095 (81.28, 46.9011) -> (81.1611, 46.9011)
  arc A5716 (80.0773, 46.549) -> (80.3019, 46.3244) centre (80.1896, 46.4367) ccw
  line L2096 (76.5511, 47.1551) -> (75.8489, 47.1551)
  line L2097 (73.8413, 47.1551) -> (73.533, 47.4634)
  arc A5717 (80.9013, 47.0207) -> (80.9509, 46.7071) centre (80.9261, 46.8639) ccw
  line L2098 (73.8396, 48.6807) -> (74.3619, 48.1584)
  line L2099 (75.4981, 50.9016) -> (74.93, 50.9016)
  arc A5718 (77.3577, 46.7286) -> (77.5823, 46.5041) centre (77.47, 46.6164) ccw
  arc A5719 (75.9096, 47.0084) -> (75.7881, 47.3018) centre (75.8488, 47.1551) ccw
  line L2100 (81.28, 44.45) -> (81.28, 46.9011)
  arc A5720 (75.4981, 47.9997) -> (75.4981, 48.3171) centre (75.4981, 48.1584) ccw
  arc A5721 (74.8177, 46.5041) -> (75.0423, 46.7286) centre (74.93, 46.6164) ccw
  arc A5722 (76.4139, 48.8496) -> (76.1893, 49.0741) centre (76.3016, 48.9619) ccw
  arc A5723 (73.7291, 47.0428) -> (73.9536, 47.2673) centre (73.8414, 47.155) ccw
  line L2101 (76.3016, 50.0981) -> (75.4981, 50.9016)
  arc A5724 (81.28, 44.6088) -> (81.28, 44.2913) centre (81.28, 44.4501) ccw
  line L2102 (79.74, 46.8863) -> (79.0911, 47.1551)
  arc A5725 (80.4158, 46.8238) -> (80.56, 46.5409) centre (80.4879, 46.6823) ccw
  arc A5726 (81.683, 47.0149) -> (81.5848, 46.7129) centre (81.6339, 46.8639) ccw
  arc A5727 (80.9752, 46.7129) -> (80.877, 47.0149) centre (80.9261, 46.8639) ccw
  arc A5728 (81.1859, 46.7443) -> (81.1362, 47.0579) centre (81.1611, 46.9011) ccw
  arc A5729 (76.6119, 47.3018) -> (76.4904, 47.0084) centre (76.5512, 47.1551) ccw
  line L2103 (81.8601, 46.7904) -> (81.6339, 46.8639)
  arc A5730 (80.2021, 46.671) -> (80.3888, 46.4141) centre (80.2954, 46.5425) ccw
  arc A5731 (81.4388, 46.9011) -> (81.1213, 46.9011) centre (81.2801, 46.9011) ccw
  line L2104 (80.6999, 46.7904) -> (80.4879, 46.6824)
  arc A5732 (81.1213, 44.45) -> (81.4388, 44.45) centre (81.2801, 44.45) ccw
  arc A5733 (81.28, 44.2913) -> (81.28, 44.6088) centre (81.28, 44.4501) ccw
  arc A5734 (77.3577, 46.5041) -> (77.5823, 46.7286) centre (77.47, 46.6164) ccw
  arc A5735 (82, 46.5409) -> (82.1442, 46.8238) centre (82.0721, 46.6824) ccw
  arc A5736 (81.28, 46.7423) -> (81.28, 47.0598) centre (81.28, 46.901) ccw
  arc A5737 (78.3889, 47.3138) -> (78.3889, 46.9963) centre (78.3889, 47.1551) ccw
  arc A5738 (76.3016, 49.3713) -> (76.3016, 49.6888) centre (76.3016, 49.5301) ccw
  line L2105 (73.533, 48.3741) -> (73.8396, 48.6807)
  arc A5739 (70.9232, 50.2033) -> (70.6057, 50.2033) centre (70.7645, 50.2033) ccw
  arc A5740 (74.7713, 49.53) -> (75.0888, 49.53) centre (74.93, 49.53) ccw
  arc A5741 (71.4057, 48.3741) -> (71.0883, 48.3741) centre (71.247, 48.3741) ccw
  arc A5742 (71.8289, 51.0433) -> (71.6044, 51.2679) centre (71.7167, 51.1556) ccw
  line L2106 (74.93, 50.9016) -> (74.93, 49.53)
  arc A5743 (74.93, 49.3712) -> (74.93, 49.6887) centre (74.93, 49.53) ccw
  arc A5744 (73.0633, 50.9968) -> (73.0633, 51.3143) centre (73.0633, 51.1556) ccw
  arc A5745 (74.2496, 48.0461) -> (74.4741, 48.2707) centre (74.3619, 48.1584) ccw
  line L2107 (71.7167, 51.1556) -> (70.7644, 50.2033)
  arc A5746 (74.3619, 51.0603) -> (74.3619, 50.7428) centre (74.3619, 50.9016) ccw
  arc A5747 (73.9519, 48.5684) -> (73.7273, 48.7929) centre (73.8396, 48.6807) ccw
  arc A5748 (75.0887, 49.53) -> (74.7712, 49.53) centre (74.93, 49.53) ccw
  arc A5749 (73.9519, 48.7929) -> (73.7273, 48.5684) centre (73.8396, 48.6807) ccw
  arc A5750 (74.3619, 48.3171) -> (74.3619, 47.9997) centre (74.3619, 48.1584) ccw
  arc A5751 (71.736, 30.4591) -> (72.0534, 30.4591) centre (71.8947, 30.4591) ccw
  line L2108 (74.93, 49.53) -> (74.93, 48.1584)
  arc A5752 (71.7167, 51.3143) -> (71.7167, 50.9968) centre (71.7167, 51.1556) ccw
  arc A5753 (74.0719, 47.3018) -> (73.9504, 47.0084) centre (74.0112, 47.1551) ccw
  arc A5754 (75.0888, 49.53) -> (74.7713, 49.53) centre (74.93, 49.53) ccw
  line L2109 (75.8489, 47.1551) -> (75.2, 46.8863)
  arc A5755 (74.7713, 49.53) -> (75.0888, 49.53) centre (74.93, 49.53) ccw
  arc A5756 (73.6453, 47.5757) -> (73.4207, 47.3512) centre (73.533, 47.4634) ccw
  line L2110 (70.7644, 48.8567) -> (71.247, 48.3741)
  arc A5757 (72.3583, 34.0433) -> (72.6758, 34.0433) centre (72.517, 34.0433) ccw
  line L2111 (71.8947, 33.0409) -> (71.8947, 30.4591)
  arc A5758 (76.3016, 49.3712) -> (76.3016, 49.6887) centre (76.3016, 49.53) ccw
  line L2112 (76.3016, 48.9619) -> (76.3016, 49.53)
  arc A5759 (73.6917, 48.3741) -> (73.3742, 48.3741) centre (73.5329, 48.3741) ccw
  arc A5760 (73.3742, 47.4634) -> (73.6917, 47.4634) centre (73.5329, 47.4634) ccw
  line L2113 (75.2, 46.8863) -> (74.93, 46.6163)
  arc A5761 (71.748, 45.8017) -> (72.0414, 45.6802) centre (71.8947, 45.7409) ccw
  arc A5762 (74.5992, 46.7397) -> (74.7207, 47.033) centre (74.6599, 46.8864) ccw
  arc A5763 (74.93, 50.7428) -> (74.93, 51.0603) centre (74.93, 50.9016) ccw
  arc A5764 (74.93, 49.3713) -> (74.93, 49.6888) centre (74.93, 49.5301) ccw
  arc A5765 (71.736, 43.1591) -> (72.0534, 43.1591) centre (71.8947, 43.1591) ccw
  line L2114 (74.93, 46.6163) -> (74.66, 46.8863)
  line L2115 (76.3016, 49.53) -> (74.93, 49.53)
  line L2116 (71.247, 46.7626) -> (71.421, 46.3425)
  line L2117 (74.3619, 50.9016) -> (73.8396, 50.3793)
  arc A5766 (74.7712, 48.1584) -> (75.0887, 48.1584) centre (74.93, 48.1584) ccw
  line L2118 (72.1634, 33.6898) -> (71.8947, 33.0409)
  line L2119 (72.517, 34.0433) -> (72.1634, 33.6898)
  line L2120 (74.93, 48.1584) -> (75.4981, 48.1584)
  arc A5767 (74.93, 49.6887) -> (74.93, 49.3712) centre (74.93, 49.53) ccw
  line L2121 (74.93, 48.1584) -> (74.93, 49.53)
  arc A5768 (74.8177, 46.7286) -> (75.0423, 46.5041) centre (74.93, 46.6164) ccw
  arc A5769 (74.7712, 49.53) -> (75.0887, 49.53) centre (74.93, 49.53) ccw
  arc A5770 (76.1893, 49.9859) -> (76.4139, 50.2104) centre (76.3016, 50.0982) ccw
  arc A5771 (74.7722, 46.9986) -> (74.5477, 46.7741) centre (74.6599, 46.8864) ccw
  arc A5772 (74.7713, 48.1584) -> (75.0888, 48.1584) centre (74.93, 48.1584) ccw
  line L2122 (74.3619, 48.1584) -> (74.93, 48.1584)
  arc A5773 (76.1428, 49.53) -> (76.4603, 49.53) centre (76.3016, 49.53) ccw
  arc A5774 (75.3859, 48.2707) -> (75.6104, 48.0461) centre (75.4981, 48.1584) ccw
  arc A5775 (73.7273, 50.4916) -> (73.9519, 50.2671) centre (73.8396, 50.3794) ccw
  arc A5776 (74.0111, 46.9963) -> (74.0111, 47.3138) centre (74.0111, 47.1551) ccw
  arc A5777 (71.8199, 45.7191) -> (72.0444, 45.9436) centre (71.9322, 45.8314) ccw
  arc A5778 (75.3123, 46.7741) -> (75.0878, 46.9986) centre (75.2, 46.8863) ccw
  arc A5779 (72.0788, 45.7706) -> (71.7855, 45.8921) centre (71.9322, 45.8314) ccw
  line L2123 (76.3016, 49.53) -> (76.3016, 50.0981)
  arc A5780 (75.0888, 50.9016) -> (74.7713, 50.9016) centre (74.93, 50.9016) ccw
  line L2124 (73.0633, 51.1556) -> (71.7167, 51.1556)
  arc A5781 (74.93, 47.9996) -> (74.93, 48.3171) centre (74.93, 48.1584) ccw
  line L2125 (71.247, 48.3741) -> (71.247, 46.7626)
  arc A5782 (71.1347, 48.2618) -> (71.3593, 48.4863) centre (71.247, 48.3741) ccw
  arc A5783 (72.0512, 33.802) -> (72.2757, 33.5775) centre (72.1635, 33.6898) ccw
  arc A5784 (73.1756, 51.2678) -> (72.9511, 51.0433) centre (73.0634, 51.1556) ccw
  arc A5785 (66.9123, 29.7697) -> (67.1368, 29.5452) centre (67.0246, 29.6575) ccw
  line L2126 (71.9322, 45.8314) -> (71.8947, 45.7409)
  arc A5786 (65.32, 29.6591) -> (65.1758, 29.3762) centre (65.2479, 29.5177) ccw
  arc A5787 (71.748, 33.1017) -> (72.0414, 32.9802) centre (71.8947, 33.041) ccw
  line L2127 (72.1634, 42.5102) -> (72.517, 42.1567)
  arc A5788 (72.6293, 33.9311) -> (72.4047, 34.1556) centre (72.517, 34.0433) ccw
  line L2128 (71.8947, 45.7409) -> (71.8947, 43.1591)
  line L2129 (71.421, 46.3425) -> (71.7425, 46.021)
  arc A5789 (70.6521, 50.3156) -> (70.8767, 50.0911) centre (70.7644, 50.2033) ccw
  arc A5790 (71.2743, 46.2818) -> (71.5677, 46.4033) centre (71.421, 46.3425) ccw
  arc A5791 (66.04, 29.4577) -> (66.04, 29.1401) centre (66.04, 29.2989) ccw
  arc A5792 (65.1546, 29.3892) -> (65.3412, 29.646) centre (65.2479, 29.5176) ccw
  arc A5793 (72.4047, 42.0444) -> (72.6293, 42.2689) centre (72.517, 42.1567) ccw
  arc A5794 (65.8962, 29.1421) -> (65.9459, 29.4557) centre (65.9211, 29.2989) ccw
  line L2130 (64.7564, 29.5701) -> (64.9496, 29.7633)
  line L2131 (71.7425, 46.021) -> (71.9322, 45.8314)
  line L2132 (65.9211, 29.2989) -> (66.04, 29.2989)
  line L2133 (74.93, 50.9016) -> (74.3619, 50.9016)
  arc A5795 (72.0414, 30.5198) -> (71.748, 30.3983) centre (71.8947, 30.4591) ccw
  arc A5796 (72.0534, 45.7409) -> (71.736, 45.7409) centre (71.8947, 45.7409) ccw
  arc A5797 (70.8767, 48.9689) -> (70.6521, 48.7444) centre (70.7644, 48.8567) ccw
  arc A5798 (71.3937, 46.8234) -> (71.1003, 46.7019) centre (71.247, 46.7627) ccw
  arc A5799 (66.9042, 29.3762) -> (66.76, 29.6591) centre (66.8321, 29.5176) ccw
  arc A5800 (66.1987, 31.75) -> (65.8812, 31.75) centre (66.04, 31.75) ccw
  line L2134 (71.8947, 43.1591) -> (72.1634, 42.5102)
  line L2135 (67.0245, 29.6574) -> (67.1928, 29.8257)
  arc A5801 (72.6758, 42.1567) -> (72.3583, 42.1567) centre (72.517, 42.1567) ccw
  line L2136 (73.8396, 50.3793) -> (73.0633, 51.1556)
  arc A5802 (72.0414, 43.2198) -> (71.748, 43.0983) centre (71.8947, 43.1591) ccw
  line L2137 (70.7644, 50.2033) -> (70.7644, 48.8567)
  line L2138 (67.1928, 29.8257) -> (67.3326, 30.0181)
  arc A5803 (64.8686, 29.6823) -> (64.6441, 29.4578) centre (64.7563, 29.57) ccw
  arc A5804 (67.1179, 29.529) -> (66.9312, 29.7859) centre (67.0246, 29.6575) ccw
  line L2139 (66.8321, 29.5176) -> (67.0245, 29.6574)
  arc A5805 (66.1988, 31.75) -> (65.8813, 31.75) centre (66.0401, 31.75) ccw
  arc A5806 (72.3101, 33.629) -> (72.0168, 33.7505) centre (72.1635, 33.6898) ccw
  arc A5807 (75.0887, 50.9016) -> (74.7712, 50.9016) centre (74.93, 50.9016) ccw
  arc A5808 (65.0619, 29.8755) -> (64.8373, 29.651) centre (64.9496, 29.7632) ccw
  arc A5809 (66.7388, 29.646) -> (66.9254, 29.3892) centre (66.8321, 29.5176) ccw
  arc A5810 (72.2757, 42.6225) -> (72.0512, 42.398) centre (72.1635, 42.5102) ccw
  arc A5811 (67.305, 29.7134) -> (67.0805, 29.9379) centre (67.1927, 29.8256) ccw
  arc A5812 (66.1589, 29.1401) -> (66.1589, 29.4577) centre (66.1589, 29.2989) ccw
  arc A5813 (71.5333, 46.4548) -> (71.3088, 46.2303) centre (71.4211, 46.3426) ccw
  arc A5814 (66.5481, 29.5511) -> (66.6922, 29.2682) centre (66.6201, 29.4096) ccw
  arc A5815 (70.6057, 48.8567) -> (70.9232, 48.8567) centre (70.7645, 48.8567) ccw
  arc A5816 (73.7273, 50.2671) -> (73.9519, 50.4916) centre (73.8396, 50.3794) ccw
  arc A5817 (64.6441, 29.6823) -> (64.8686, 29.4578) centre (64.7563, 29.5701) ccw
  arc A5818 (65.5089, 29.5606) -> (65.4108, 29.2586) centre (65.4599, 29.4096) ccw
  arc A5819 (71.0883, 46.7626) -> (71.4057, 46.7626) centre (71.247, 46.7626) ccw
  arc A5820 (74.93, 49.6888) -> (74.93, 49.3713) centre (74.93, 49.5301) ccw
  arc A5821 (71.8548, 46.1333) -> (71.6303, 45.9088) centre (71.7426, 46.0211) ccw
  arc A5822 (72.0168, 42.4495) -> (72.3101, 42.571) centre (72.1635, 42.5102) ccw
  line L2140 (74.93, 49.53) -> (74.93, 50.9016)
  arc A5823 (65.1312, 28.9707) -> (65.3557, 29.1953) centre (65.2434, 29.083) ccw
  arc A5824 (74.4741, 50.7893) -> (74.2496, 51.0139) centre (74.3619, 50.9016) ccw
  arc A5825 (65.7109, 29.4929) -> (65.6613, 29.1793) centre (65.6861, 29.3361) ccw
  line L2141 (72.517, 42.1567) -> (72.517, 34.0433)
  arc A5826 (71.6303, 45.9088) -> (71.8548, 46.1333) centre (71.7426, 46.0211) ccw
  arc A5827 (64.9432, 29.5452) -> (65.1677, 29.7697) centre (65.0555, 29.6575) ccw
  arc A5828 (65.8812, 29.2989) -> (66.1987, 29.2989) centre (66.04, 29.2989) ccw
  line L2142 (65.4599, 29.4096) -> (65.6861, 29.3361)
  arc A5829 (65.8812, 31.75) -> (66.1987, 31.75) centre (66.04, 31.75) ccw
  arc A5830 (71.9166, 28.9242) -> (71.9166, 29.2417) centre (71.9166, 29.083) ccw
  arc A5831 (67.474, 33.554) -> (67.1911, 33.4098) centre (67.3326, 33.4819) ccw
  line L2143 (65.6861, 29.3361) -> (65.9211, 29.2989)
  line L2144 (65.2434, 29.083) -> (64.7564, 29.5701)
  arc A5832 (65.3878, 29.2682) -> (65.5319, 29.5511) centre (65.4599, 29.4097) ccw
  arc A5833 (66.04, 31.9087) -> (66.04, 31.5912) centre (66.04, 31.75) ccw
  arc A5834 (66.1341, 29.4557) -> (66.1838, 29.1421) centre (66.159, 29.2989) ccw
  arc A5835 (66.9254, 34.1108) -> (66.7388, 33.8539) centre (66.8321, 33.9824) ccw
  arc A5836 (67.5916, 33.319) -> (67.2896, 33.2209) centre (67.4406, 33.27) ccw
  arc A5837 (67.5513, 31.5913) -> (67.5513, 31.9088) centre (67.5513, 31.7501) ccw
  line L2145 (66.04, 29.2989) -> (66.1589, 29.2989)
  line L2146 (66.6201, 34.0904) -> (66.3939, 34.1639)
  line L2147 (66.04, 34.2011) -> (65.9211, 34.2011)
  arc A5838 (65.1488, 29.7859) -> (64.9621, 29.529) centre (65.0555, 29.6575) ccw
  line L2148 (67.0245, 33.8426) -> (66.8321, 33.9824)
  line L2149 (66.04, 31.75) -> (67.5513, 31.75)
  line L2150 (67.5141, 30.4563) -> (67.5513, 30.6913)
  arc A5839 (66.04, 31.5913) -> (66.04, 31.9088) centre (66.04, 31.7501) ccw
  arc A5840 (67.3631, 32.9946) -> (67.6651, 33.0928) centre (67.5141, 33.0437) ccw
  arc A5841 (65.9211, 29.4577) -> (65.9211, 29.1401) centre (65.9211, 29.2989) ccw
  arc A5842 (66.4187, 29.1793) -> (66.3691, 29.4929) centre (66.3939, 29.3361) ccw
  arc A5843 (72.0168, 29.7495) -> (72.3101, 29.871) centre (72.1635, 29.8103) ccw
  arc A5844 (72.2757, 29.9225) -> (72.0512, 29.698) centre (72.1635, 29.8102) ccw
  line L2151 (66.6201, 29.4096) -> (66.8321, 29.5176)
  arc A5845 (67.2041, 33.3886) -> (67.461, 33.5752) centre (67.3325, 33.4819) ccw
  arc A5846 (67.3945, 32.7839) -> (67.7081, 32.8336) centre (67.5513, 32.8088) ccw
  line L2152 (67.3326, 30.0181) -> (67.4406, 30.2301)
  arc A5847 (67.2896, 30.2791) -> (67.5916, 30.181) centre (67.4406, 30.2301) ccw
  arc A5848 (66.5711, 33.9394) -> (66.6692, 34.2414) centre (66.6201, 34.0904) ccw
  line L2153 (71.9166, 29.083) -> (65.2434, 29.083)
  arc A5849 (65.8813, 31.75) -> (66.1988, 31.75) centre (66.0401, 31.75) ccw
  arc A5850 (67.0805, 33.5621) -> (67.305, 33.7866) centre (67.1927, 33.6744) ccw
  arc A5851 (72.5159, 29.4578) -> (72.2914, 29.6823) centre (72.4036, 29.5701) ccw
  arc A5852 (71.8043, 29.1953) -> (72.0288, 28.9707) centre (71.9166, 29.083) ccw
  line L2154 (67.5513, 31.75) -> (66.04, 31.75)
  line L2155 (66.04, 29.2989) -> (66.04, 31.75)
  line L2156 (64.9496, 29.7633) -> (65.0555, 29.6574)
  line L2157 (72.1634, 29.8102) -> (72.4036, 29.5701)
  line L2158 (66.1589, 29.2989) -> (66.3939, 29.3361)
  line L2159 (66.04, 34.2011) -> (66.04, 31.75)
  arc A5853 (67.461, 29.9248) -> (67.2041, 30.1114) centre (67.3325, 30.0181) ccw
  line L2160 (67.5513, 31.75) -> (67.5513, 32.8087)
  arc A5854 (66.04, 31.5912) -> (66.04, 31.9087) centre (66.04, 31.75) ccw
  line L2161 (71.8947, 30.4591) -> (72.1634, 29.8102)
  arc A5855 (65.8813, 29.2989) -> (66.1988, 29.2989) centre (66.0401, 29.2989) ccw
  line L2162 (65.0555, 29.6574) -> (65.2479, 29.5176)
  arc A5856 (72.2914, 29.4578) -> (72.5159, 29.6823) centre (72.4036, 29.57) ccw
  line L2163 (65.2479, 29.5176) -> (65.4599, 29.4096)
  arc A5857 (66.3448, 29.4871) -> (66.443, 29.1851) centre (66.3939, 29.3361) ccw
  line L2164 (72.4036, 29.5701) -> (71.9166, 29.083)
  arc A5858 (66.6692, 29.2586) -> (66.5711, 29.5606) centre (66.6201, 29.4096) ccw
  line L2165 (66.04, 31.75) -> (66.04, 29.2989)
  line L2166 (66.3939, 29.3361) -> (66.6201, 29.4096)
  arc A5859 (65.637, 29.1851) -> (65.7352, 29.4871) centre (65.6861, 29.3361) ccw
  arc A5860 (65.0619, 29.651) -> (64.8373, 29.8755) centre (64.9496, 29.7632) ccw
  arc A5861 (66.04, 34.3598) -> (66.04, 34.0423) centre (66.04, 34.2011) ccw
  arc A5862 (72.0534, 33.0409) -> (71.736, 33.0409) centre (71.8947, 33.0409) ccw
  arc A5863 (66.04, 29.1401) -> (66.04, 29.4577) centre (66.04, 29.2989) ccw
  arc A5864 (65.2434, 29.2417) -> (65.2434, 28.9242) centre (65.2434, 29.083) ccw
  arc A5865 (66.1838, 34.3579) -> (66.1341, 34.0443) centre (66.159, 34.2011) ccw
  arc A5866 (66.04, 31.9088) -> (66.04, 31.5913) centre (66.04, 31.7501) ccw
  arc A5867 (67.582, 30.158) -> (67.2991, 30.3021) centre (67.4406, 30.2301) ccw
  arc A5868 (66.1988, 31.75) -> (65.8813, 31.75) centre (66.0401, 31.75) ccw
  arc A5869 (66.3691, 34.0071) -> (66.4187, 34.3207) centre (66.3939, 34.1639) ccw
  arc A5870 (65.8813, 31.75) -> (66.1988, 31.75) centre (66.0401, 31.75) ccw
  line L2167 (60.6089, 29.0449) -> (61.3111, 29.0449)
  arc A5871 (59.048, 33.1017) -> (59.3414, 32.9802) centre (59.1947, 33.041) ccw
  arc A5872 (67.6651, 30.4072) -> (67.3631, 30.5054) centre (67.5141, 30.4563) ccw
  arc A5873 (67.1911, 30.0902) -> (67.474, 29.946) centre (67.3326, 30.0181) ccw
  arc A5874 (67.0643, 29.919) -> (67.3212, 29.7323) centre (67.1928, 29.8257) ccw
  line L2168 (66.3939, 34.1639) -> (66.1589, 34.2011)
  arc A5875 (67.2991, 33.1979) -> (67.582, 33.342) centre (67.4406, 33.27) ccw
  arc A5876 (65.9459, 34.0443) -> (65.8962, 34.3579) centre (65.9211, 34.2011) ccw
  arc A5877 (67.3925, 30.6913) -> (67.71, 30.6913) centre (67.5513, 30.6913) ccw
  arc A5878 (66.04, 31.9087) -> (66.04, 31.5912) centre (66.04, 31.75) ccw
  arc A5879 (67.3573, 30.4811) -> (67.6709, 30.4315) centre (67.5141, 30.4563) ccw
  line L2169 (67.1928, 33.6743) -> (67.0245, 33.8426)
  arc A5880 (66.6922, 34.2318) -> (66.5481, 33.9489) centre (66.6201, 34.0904) ccw
  arc A5881 (67.5513, 31.5912) -> (67.5513, 31.9087) centre (67.5513, 31.75) ccw
  arc A5882 (67.6709, 33.0685) -> (67.3573, 33.0189) centre (67.5141, 33.0437) ccw
  arc A5883 (66.1988, 34.2011) -> (65.8813, 34.2011) centre (66.0401, 34.2011) ccw
  arc A5884 (66.9312, 33.7141) -> (67.1179, 33.971) centre (67.0245, 33.8426) ccw
  line L2170 (67.4406, 30.2301) -> (67.5141, 30.4563)
  arc A5885 (67.71, 31.75) -> (67.3925, 31.75) centre (67.5513, 31.75) ccw
  line L2171 (67.4406, 33.2699) -> (67.3326, 33.4819)
  arc A5886 (65.6613, 34.3207) -> (65.7109, 34.0071) centre (65.6861, 34.1639) ccw
  line L2172 (66.8321, 33.9824) -> (66.6201, 34.0904)
  arc A5887 (66.76, 33.8409) -> (66.9042, 34.1238) centre (66.8321, 33.9824) ccw
  arc A5888 (64.4392, 34.0397) -> (64.5607, 34.333) centre (64.4999, 34.1864) ccw
  arc A5889 (59.8993, 34.333) -> (60.0208, 34.0397) centre (59.9601, 34.1864) ccw
  arc A5890 (67.3925, 31.75) -> (67.71, 31.75) centre (67.5513, 31.75) ccw
  arc A5891 (66.04, 31.9088) -> (66.04, 31.5913) centre (66.04, 31.7501) ccw
  arc A5892 (66.1589, 34.0423) -> (66.1589, 34.3598) centre (66.1589, 34.2011) ccw
  arc A5893 (67.7081, 30.6664) -> (67.3945, 30.7161) centre (67.5513, 30.6912) ccw
  line L2173 (66.04, 31.75) -> (66.04, 34.2011)
  line L2174 (67.5141, 33.0437) -> (67.4406, 33.2699)
  arc A5894 (66.443, 34.3149) -> (66.3448, 34.0129) centre (66.3939, 34.1639) ccw
  arc A5895 (67.1368, 33.9548) -> (66.9123, 33.7303) centre (67.0246, 33.8425) ccw
  arc A5896 (66.1987, 34.2011) -> (65.8812, 34.2011) centre (66.04, 34.2011) ccw